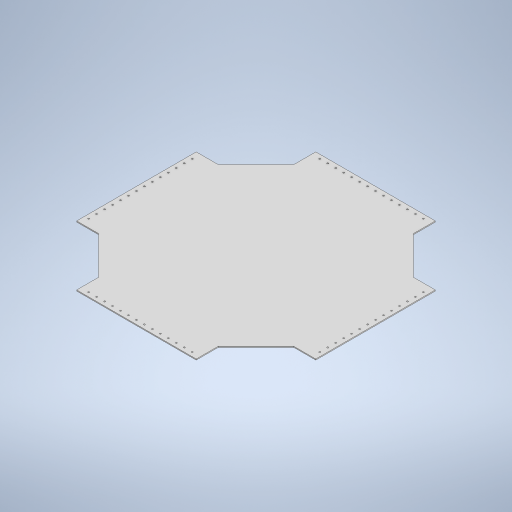
# Autodesk Inventor part: Base Plate V1.2
Saved by Autodesk Inventor 2023 (Build 270158000, 158)
## iProperties
Created: 2023-01-11
Part Number: Base Plate V1.2
Material: Generic
Document SubType Name: Modeling
Designer: Gabriel - T3 CAD
Density: 1 g/cm^3
Appearance: Default
Author: Gabriel - T3 CAD
Autodesk Inventor part; units mm, degrees
ref_plane "YZ Plane" through (0, 0, 0) normal (1, 0, 0) x (0, 1, 0)
ref_plane "XZ Plane" through (0, 0, 0) normal (0, 1, 0) x (-1, 0, 0)
ref_plane "XY Plane" through (0, 0, 0) normal (0, 0, 1) x (1, 0, 0)
sketch "Sketch1" plane through (0, 0, 0) normal (0, 1, 0) x (-1, 0, 0)
  line L0 (0, 0) -> (762, 0)
  line L1 (762, 0) -> (762, 762)
  line L2 (762, 762) -> (0, 762)
  line L3 (0, 762) -> (0, 0)
  line L4 (0, 0) -> (190.5, 0)
  line L5 (190.5, 0) -> (190.5, 69.85)
  line L6 (190.5, 69.85) -> (0, 69.85)
  line L7 (0, 69.85) -> (0, 0)
  line L8 (0, 0) -> (69.85, 0)
  line L9 (69.85, 0) -> (69.85, 190.5)
  line L10 (69.85, 190.5) -> (0, 190.5)
  line L11 (0, 190.5) -> (0, 0)
  line L12 (69.85, 190.5) -> (190.5, 69.85)
  line L13 (381, 0) -> (381, 762)
  line L14 (0, 381) -> (762, 381)
  line L15 (190.5, 762) -> (190.5, 692.15)
  line L16 (190.5, 692.15) -> (0, 692.15)
  line L17 (69.85, 762) -> (69.85, 571.5)
  line L18 (69.85, 571.5) -> (0, 571.5)
  line L19 (69.85, 571.5) -> (190.5, 692.15)
  line L20 (571.5, 0) -> (571.5, 69.85)
  line L21 (571.5, 69.85) -> (762, 69.85)
  line L22 (692.15, 0) -> (692.15, 190.5)
  line L23 (692.15, 190.5) -> (762, 190.5)
  line L24 (692.15, 190.5) -> (571.5, 69.85)
  line L25 (571.5, 692.15) -> (762, 692.15)
  line L26 (692.15, 571.5) -> (571.5, 692.15)
  line L27 (692.15, 762) -> (692.15, 571.5)
  line L28 (571.5, 762) -> (571.5, 692.15)
  line L29 (692.15, 571.5) -> (762, 571.5)
  circle A0 centre (749.3, 749.3) radius 2.3812
  circle A1 centre (749.3, 723.9) radius 2.3812
  circle A2 centre (749.3, 698.5) radius 2.3812
  circle A3 centre (749.3, 673.1) radius 2.3812
  circle A4 centre (749.3, 647.7) radius 2.3812
  circle A5 centre (749.3, 622.3) radius 2.3812
  circle A6 centre (749.3, 596.9) radius 2.3812
  circle A7 centre (749.3, 571.5) radius 2.3812
  circle A8 centre (749.3, 546.1) radius 2.3812
  circle A9 centre (749.3, 520.7) radius 2.3812
  circle A10 centre (749.3, 495.3) radius 2.3812
  circle A11 centre (749.3, 469.9) radius 2.3812
  circle A12 centre (749.3, 444.5) radius 2.3812
  circle A13 centre (749.3, 419.1) radius 2.3812
  circle A14 centre (749.3, 393.7) radius 2.3812
  circle A15 centre (749.3, 368.3) radius 2.3812
  circle A16 centre (749.3, 342.9) radius 2.3812
  circle A17 centre (749.3, 317.5) radius 2.3812
  circle A18 centre (749.3, 292.1) radius 2.3812
  circle A19 centre (749.3, 266.7) radius 2.3812
  circle A20 centre (749.3, 241.3) radius 2.3812
  circle A21 centre (749.3, 215.9) radius 2.3812
  circle A22 centre (749.3, 190.5) radius 2.3812
  circle A23 centre (749.3, 165.1) radius 2.3812
  circle A24 centre (749.3, 139.7) radius 2.3812
  circle A25 centre (749.3, 114.3) radius 2.3812
  circle A26 centre (749.3, 88.9) radius 2.3812
  circle A27 centre (749.3, 63.5) radius 2.3812
  circle A28 centre (749.3, 38.1) radius 2.3812
  circle A29 centre (749.3, 12.7) radius 2.3812
  circle A30 centre (12.7, 749.3) radius 2.3812
  circle A31 centre (12.7, 723.9) radius 2.3812
  circle A32 centre (12.7, 698.5) radius 2.3812
  circle A33 centre (12.7, 673.1) radius 2.3812
  circle A34 centre (12.7, 647.7) radius 2.3812
  circle A35 centre (12.7, 622.3) radius 2.3812
  circle A36 centre (12.7, 596.9) radius 2.3812
  circle A37 centre (12.7, 571.5) radius 2.3812
  circle A38 centre (12.7, 546.1) radius 2.3812
  circle A39 centre (12.7, 520.7) radius 2.3812
  circle A40 centre (12.7, 495.3) radius 2.3812
  circle A41 centre (12.7, 469.9) radius 2.3812
  circle A42 centre (12.7, 444.5) radius 2.3812
  circle A43 centre (12.7, 419.1) radius 2.3812
  circle A44 centre (12.7, 393.7) radius 2.3812
  circle A45 centre (12.7, 368.3) radius 2.3812
  circle A46 centre (12.7, 342.9) radius 2.3812
  circle A47 centre (12.7, 317.5) radius 2.3812
  circle A48 centre (12.7, 292.1) radius 2.3812
  circle A49 centre (12.7, 266.7) radius 2.3812
  circle A50 centre (12.7, 241.3) radius 2.3812
  circle A51 centre (12.7, 215.9) radius 2.3812
  circle A52 centre (12.7, 190.5) radius 2.3812
  circle A53 centre (12.7, 165.1) radius 2.3812
  circle A54 centre (12.7, 139.7) radius 2.3812
  circle A55 centre (12.7, 114.3) radius 2.3812
  circle A56 centre (12.7, 88.9) radius 2.3812
  circle A57 centre (12.7, 63.5) radius 2.3812
  circle A58 centre (12.7, 38.1) radius 2.3812
  circle A59 centre (12.7, 12.7) radius 2.3812
  circle A60 centre (723.9, 749.3) radius 2.3812
  circle A61 centre (698.5, 749.3) radius 2.3812
  circle A62 centre (673.1, 749.3) radius 2.3812
  circle A63 centre (647.7, 749.3) radius 2.3812
  circle A64 centre (622.3, 749.3) radius 2.3812
  circle A65 centre (596.9, 749.3) radius 2.3812
  circle A66 centre (571.5, 749.3) radius 2.3812
  circle A67 centre (546.1, 749.3) radius 2.3812
  circle A68 centre (520.7, 749.3) radius 2.3812
  circle A69 centre (495.3, 749.3) radius 2.3812
  circle A70 centre (469.9, 749.3) radius 2.3812
  circle A71 centre (444.5, 749.3) radius 2.3812
  circle A72 centre (419.1, 749.3) radius 2.3812
  circle A73 centre (393.7, 749.3) radius 2.3812
  circle A74 centre (368.3, 749.3) radius 2.3812
  circle A75 centre (342.9, 749.3) radius 2.3812
  circle A76 centre (317.5, 749.3) radius 2.3812
  circle A77 centre (292.1, 749.3) radius 2.3812
  circle A78 centre (266.7, 749.3) radius 2.3812
  circle A79 centre (241.3, 749.3) radius 2.3812
  circle A80 centre (215.9, 749.3) radius 2.3812
  circle A81 centre (190.5, 749.3) radius 2.3812
  circle A82 centre (165.1, 749.3) radius 2.3812
  circle A83 centre (139.7, 749.3) radius 2.3812
  circle A84 centre (114.3, 749.3) radius 2.3812
  circle A85 centre (88.9, 749.3) radius 2.3812
  circle A86 centre (63.5, 749.3) radius 2.3812
  circle A87 centre (38.1, 749.3) radius 2.3812
  circle A88 centre (12.7, 749.3) radius 2.3812
  circle A89 centre (749.3, 12.7) radius 2.3812
  circle A90 centre (723.9, 12.7) radius 2.3812
  circle A91 centre (698.5, 12.7) radius 2.3812
  circle A92 centre (673.1, 12.7) radius 2.3812
  circle A93 centre (647.7, 12.7) radius 2.3812
  circle A94 centre (622.3, 12.7) radius 2.3812
  circle A95 centre (596.9, 12.7) radius 2.3812
  circle A96 centre (571.5, 12.7) radius 2.3812
  circle A97 centre (546.1, 12.7) radius 2.3812
  circle A98 centre (520.7, 12.7) radius 2.3812
  circle A99 centre (495.3, 12.7) radius 2.3812
  circle A100 centre (469.9, 12.7) radius 2.3812
  circle A101 centre (444.5, 12.7) radius 2.3812
  circle A102 centre (419.1, 12.7) radius 2.3812
  circle A103 centre (393.7, 12.7) radius 2.3812
  circle A104 centre (368.3, 12.7) radius 2.3812
  circle A105 centre (342.9, 12.7) radius 2.3812
  circle A106 centre (317.5, 12.7) radius 2.3812
  circle A107 centre (292.1, 12.7) radius 2.3812
  circle A108 centre (266.7, 12.7) radius 2.3812
  circle A109 centre (241.3, 12.7) radius 2.3812
  circle A110 centre (215.9, 12.7) radius 2.3812
  circle A111 centre (190.5, 12.7) radius 2.3812
  circle A112 centre (165.1, 12.7) radius 2.3812
  circle A113 centre (139.7, 12.7) radius 2.3812
  circle A114 centre (114.3, 12.7) radius 2.3812
  circle A115 centre (88.9, 12.7) radius 2.3812
  circle A116 centre (63.5, 12.7) radius 2.3812
  circle A117 centre (38.1, 12.7) radius 2.3812
  circle A118 centre (12.7, 12.7) radius 2.3812
  dimension "d0" = 762
  dimension "d1" = 762
  dimension "d2" = 190.5
  dimension "d3" = 69.85
  dimension "d4" = 69.85
  dimension "d5" = 190.5
  dimension "d29" = 12.7
  dimension "d30" = 12.7
  dimension "d31" = 4.7625
  dimension "d34" = 25.4
  dimension "d37" = 736.6
  dimension "d42" = 25.4
  dimension "d45" = 736.6
  constraints: 119 centre point, 60 end point, 18 symmetric about line, 6 parallel, 5 horizontal, 4 midpoint, 3 perpendicular, 2 vertical, 236 other
  measures "d0" distance of L2.end L1.end
  measures "d1" distance of L1.end L0.end
  measures "d2" distance of L6.end L5.end
  measures "d3" distance of L5.end L4.end
  measures "d4" distance of L10.end L9.end
  measures "d5" distance of L9.end L8.end
  measures "d29" distance from line of L2 A0.centre
  measures "d30" distance from line of L1 A0.centre
  measures "d31" diameter of A0
  measures "d34" distance of A0.centre A1.centre
  measures "d37" distance of A0.centre A30.centre
  measures "d42" distance of A0.centre A60.centre
  measures "d45" distance of A0.centre A89.centre
extrude "Extrusion1" add sketch "Sketch1" along normal blind 3.175 contours L5 A111 L12 L10 A52 L3 L14 L13 L0 | L13 L14 L1 L23 A22 L24 L20 A96 L0 | L5 A111 | L3 L18 A37 L19 L15 A81 L2 L13 L14 | A52 L10 | L13 L2 L28 A66 L26 L29 A7 L1 L14 | A96 L20 | L18 A37 | L28 A66 | A81 L15 | L23 A22 | A7 L29 picked at (191.2937, 12.7) picked at (13.1509, 191.1532) picked at (570.7578, 12.4185) picked at (12.2491, 570.8468) picked at (570.7578, 749.5815) picked at (191.6271, 749.4766) picked at (749.3957, 191.6679) picked at (749.5815, 570.7578)
body "Solid1"
